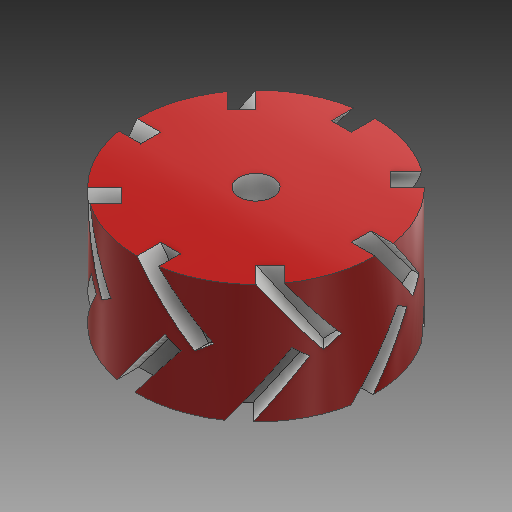
# Autodesk Inventor part: Wheel
Saved by Autodesk Inventor 2018 (Build 220112000, 112)
## iProperties
Created: 2018-10-25
Part Number: Wheel
Material: Generic
Document SubType Name: Modeling
Designer: iki
Density: 1 g/cm^3
Appearance: Default
Mass: 9.62186 g
Surface Area: 36.9516 cm^2
Volume: 9.62186 cm^3
Author: iki
Autodesk Inventor part; units mm, degrees
ref_plane "YZ Plane" through (0, 0, 0) normal (1, 0, 0) x (0, 1, 0)
ref_plane "XZ Plane" through (0, 0, 0) normal (0, 1, 0) x (-1, 0, 0)
sketch "Sketch1" plane through (0, 0, 0) normal (0, 0, 1) x (1, 0, 0)
  circle A0 centre (0, 0) radius 2.15
  circle A1 centre (0, 0) radius 15
  dimension "d0" = 4.3
  dimension "d1" = 30
  constraints: 2 centre point, 2 coincident
  measures "d0" diameter of A0
  measures "d1" diameter of A1
extrude "Extrusion1" add sketch "Sketch1" along normal blind 15
sketch "Sketch3" plane through (0, 0, 15) normal (0, 0, 1) x (1, 0, 0)
  point P0 (0, 0)
  point P1 (0, 15)
ref_plane "Work Plane1" through (0, 15, 15) normal (0, 1, 0) x (-1, 0, 0)
sketch "Sketch4" plane through (0, 15, 15) normal (0, 1, 0) x (-1, 0, 0)
  line L0 (15, 0) -> (-15, 0) projected
  line L1 (0, 0) -> (1.5987, 1.2017)
  line L2 (1.5987, 1.2017) -> (7.6071, -6.792)
  line L3 (7.6071, -6.792) -> (6.0084, -7.9937)
  line L4 (6.0084, -7.9937) -> (0, 0)
  line L5 (3.1858, -7.1278) -> (4.7814, -8.3336)
  line L6 (4.7814, -8.3336) -> (-1.2479, -16.3116)
  line L7 (-1.2479, -16.3116) -> (-2.8435, -15.1057)
  line L8 (-2.8435, -15.1057) -> (3.1858, -7.1278)
  point P0 (0, -15)
  dimension "d8" = 2
  dimension "d9" = 10
  dimension "d10" = 2
  dimension "d11" = 10
  constraints: 16 end point, 4 parallel, 2 perpendicular
  measures "d8" distance of L2.end L3.end
  measures "d9" distance of L1.end L2.end
  measures "d10" distance of L7.start L7.end
  measures "d11" distance of L6.start L7.start
extrude "Extrusion3" cut sketch "Sketch4" against normal blind 3
pattern_circular "Circular Pattern1" count 8 over 360 about axis through (0, 0, 0) along (0, 0, 1) of "Extrusion3"
body "Solid1"
